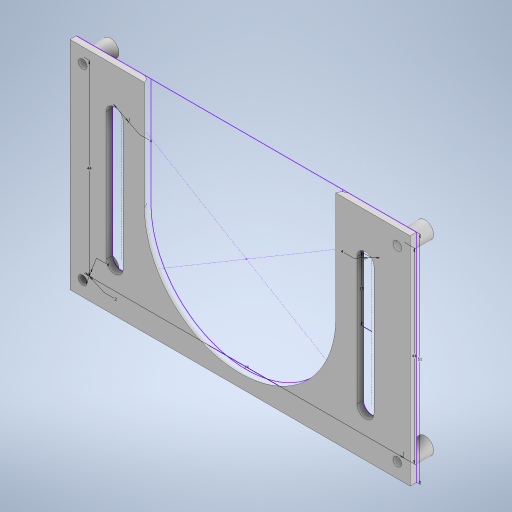
# Autodesk Inventor part: FrontHolder
Saved by Autodesk Inventor 2024 (Build 280153000, 153)
## iProperties
Created: 2025-05-21
Part Number: FrontHolder
Material: Ogólny
Document SubType Name: Modeling
Designer: Victoria
Density: 1 g/cm^3
Appearance: Domyślna
Author: Victoria
Autodesk Inventor part; units mm, degrees
ref_plane "YZ Plane" through (0, 0, 0) normal (1, 0, 0) x (0, 1, 0)
ref_plane "XZ Plane" through (0, 0, 0) normal (0, 1, 0) x (-1, 0, 0)
ref_plane "XY Plane" through (0, 0, 0) normal (0, 0, 1) x (1, 0, 0)
sketch "Szkic1" plane through (0, 0, 0) normal (0, 0, 1) x (1, 0, 0)
  line L0 (-40, -25.5) -> (40, -25.5)
  line L1 (40, -25.5) -> (40, 25.5)
  line L2 (40, 25.5) -> (-40, 25.5)
  line L3 (-40, 25.5) -> (-40, -25.5)
  line L4 (22.5, 0) -> (22.5, 25.5)
  line L5 (22.5, 25.5) -> (-22.5, 25.5)
  line L6 (-22.5, -25.5) -> (22.5, -25.5)
  line L7 (-29.5, -15) -> (-29.5, 15) construction
  line L8 (-27.5, -15) -> (-27.5, 15)
  line L9 (-31.5, 15) -> (-31.5, -15)
  arc A0 (-31.5, -15) -> (-27.5, -15) centre (-29.5, -15) ccw
  arc A1 (-27.5, 15) -> (-31.5, 15) centre (-29.5, 15) ccw
  line L10 (29.5, -15) -> (29.5, 15) construction
  line L11 (31.5, -15) -> (31.5, 15)
  line L12 (27.5, 15) -> (27.5, -15)
  arc A2 (27.5, -15) -> (31.5, -15) centre (29.5, -15) ccw
  arc A3 (31.5, 15) -> (27.5, 15) centre (29.5, 15) ccw
  line L13 (27.5, 0) -> (29.5, 0)
  arc A4 (-22.5, 0) -> (22.5, 0) centre (0, 0) ccw
  line L14 (-22.5, 25.5) -> (-22.5, 0)
  line L15 (37, -22) -> (-37, -22)
  line L16 (-37, -22) -> (-37, 22)
  line L17 (-37, 22) -> (37, -22) construction
  line L18 (37, 22) -> (-37, -22) construction
  circle A5 centre (-37, -22) radius 1
  circle A6 centre (-37, -22) radius 2
  circle A7 centre (37, -22) radius 2
  circle A8 centre (37, -22) radius 1
  circle A9 centre (-37, 22) radius 2
  circle A10 centre (-37, 22) radius 1
  circle A11 centre (37, 22) radius 2
  circle A12 centre (37, 22) radius 1
  dimension "d1" = 51
  dimension "d14" = 4
  dimension "d15" = 15
  dimension "d16" = 4
  dimension "d26" = 44
  dimension "d27" = 2
  dimension "d28" = 4
  dimension "d31" = 74
  dimension "d34" = 44
  constraints: 42 end point, 13 centre point, 10 point on circle, 8 tangent, 7 parallel, 5 coincident, 4 midpoint, 2 horizontal, 2 perpendicular, 2 vertical, 12 other
  measures "d1" distance of L1.end L0.end
  measures "d14" diameter of A1
  measures "d15" distance of L13.end L10.end
  measures "d16" diameter of A3
  measures "d26" distance of L18.start L15.start
  measures "d27" diameter of A5
  measures "d28" diameter of A6
  measures "d31" distance of A6.centre A7.centre
  measures "d34" distance of A6.centre A9.centre
extrude "Wyciągnięcie proste1" add sketch "Szkic1" along normal blind 1.5 contours L3 L2 L14 A4 L4 L1 L0 | A6 L16 A5 L15 | L15 A5 L16 A6 | A7 | A9 | A11
extrude "Wyciągnięcie proste2" add sketch "Szkic1" against normal blind 5 contours A6 L16 A5 L15 | L15 A5 L16 A6 | A7 | A9 | A11
fillet "Zaokrąglenie1" radius 2 3 edges at (-22.5, 12.75, 0) (22.5, 12.75, 0) (0, -22.5, 0)
